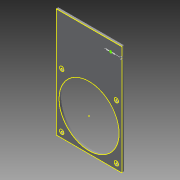
# Autodesk Inventor part: base_usb3
Saved by Autodesk Inventor 2014 (Build 180170000, 170)
## iProperties
Created: 2015-04-20
Part Number: base_usb3
Material: Generic
Document SubType Name: Modeling
Designer: Sousaadm
Density: 1 g/cm^3
Appearance: Default
Author: Sousaadm
Autodesk Inventor part; units mm, degrees
ref_plane "YZ Plane" through (0, 0, 0) normal (1, 0, 0) x (0, 1, 0)
ref_plane "XZ Plane" through (0, 0, 0) normal (0, 1, 0) x (-1, 0, 0)
ref_plane "XY Plane" through (0, 0, 0) normal (0, 0, 1) x (1, 0, 0)
sketch "Sketch1" plane through (0, 0, 0) normal (0, 1, 0) x (-1, 0, 0)
  line L0 (0, 0) -> (-60, 0)
  line L1 (-60, 0) -> (-60, 100)
  line L2 (-60, 100) -> (0, 100)
  line L3 (0, 100) -> (0, 0)
  dimension "d0" = 100
  dimension "d1" = 60
  constraints: 8 end point, 2 parallel, 1 horizontal, 1 perpendicular
  measures "d0" distance of L2.end L0.start
  measures "d1" distance of L1.end L2.end
extrude "Extrusion1" add sketch "Sketch1" along normal blind 2
sketch "Sketch2" plane through (0, 0, 0) normal (0, -1, 0) x (1, 0, 0)
  line L0 (60, 0) -> (60, 100) projected
  line L1 (60, 100) -> (0, 100) projected
  circle A0 centre (55, 55) radius 2
  circle A1 centre (5, 55) radius 2
  circle A2 centre (55, 5) radius 2
  circle A3 centre (5, 5) radius 2
  line L2 (0, 0) -> (60, 0) projected
  dimension "d7" = 4
  dimension "d40" = 5
  dimension "d44" = 50
  dimension "d47" = 50
  dimension "d56" = 55
  constraints: 4 centre point, 1 horizontal, 1 vertical, 6 other
  measures "d7" diameter of A0
  measures "d40" distance from line of L0 A0.centre
  measures "d44" distance of A0.centre A1.centre
  measures "d47" distance of A0.centre A2.centre
  measures "d56" distance from line of L2 A0.centre
extrude "Extrusion2" cut sketch "Sketch2" against normal through all
sketch "Sketch4" plane through (0, 0, 0) normal (0, -1, 0) x (1, 0, 0)
  line L0 (0, 0) -> (60, 0) projected
  line L1 (60, 0) -> (60, 100) projected
  circle A0 centre (30, 30) radius 27.5
  dimension "d50" = 55
  dimension "d52" = 30
  dimension "d53" = 30
  constraints: 1 centre point
  measures "d50" diameter of A0
  measures "d52" distance from line of L1 A0.centre
  measures "d53" distance from line of L0 A0.centre
extrude "Extrusion4" cut sketch "Sketch4" against normal through all
sketch "Sketch5" plane through (0, 0, 0) normal (0, -1, 0) x (1, 0, 0)
  circle A0 centre (30, 30) radius 27.5 projected
  circle A1 centre (55, 5) radius 2 projected
  circle A2 centre (55, 55) radius 2 projected
  circle A3 centre (5, 55) radius 2 projected
  circle A4 centre (5, 5) radius 2 projected
  line L0 (0, 0) -> (60, 0) projected
  line L1 (60, 0) -> (60, 100) projected
  line L2 (60, 100) -> (0, 100) projected
  line L3 (0, 100) -> (0, 0) projected
  circle A5 centre (49.802, 90.775) radius 1
  dimension "d57" = 2
  constraints: 1 centre point
  measures "d57" diameter of A5
equation "\"d52\" = 0.5 * d1"
body "Solid1"
